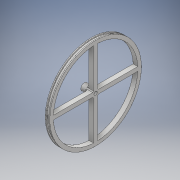
# Autodesk Inventor part: mtv_pushingWheel_2-25
Saved by Autodesk Inventor 2018 (Build 220112000, 112)
## iProperties
Created: 2019-02-07
Part Number: mtv_pushingWheel_2-25
Material: Generic
Document SubType Name: Modeling
Designer: Aditya Kendre
Density: 1 g/cm^3
Appearance: Default
Author: Aditya Kendre
Autodesk Inventor part; units mm, degrees
ref_plane "YZ Plane" through (0, 0, 0) normal (1, 0, 0) x (0, 1, 0)
ref_plane "XZ Plane" through (0, 0, 0) normal (0, 1, 0) x (-1, 0, 0)
ref_plane "XY Plane" through (0, 0, 0) normal (0, 0, 1) x (1, 0, 0)
sketch "Sketch1" plane through (0, 0, 0) normal (1, 0, 0) x (0, 1, 0)
  circle A0 centre (0, 0) radius 44
  dimension "d0" = 88
  constraints: 1 centre point, 1 coincident
  measures "d0" diameter of A0
extrude "Extrusion1" add sketch "Sketch1" along normal blind 3.5
sketch "Sketch2" plane through (3.5, 0, 0) normal (1, 0, 0) x (0, 0, -1)
  circle A0 centre (0, 0) radius 45
  dimension "d3" = 90
  constraints: 1 centre point, 1 coincident
  measures "d3" diameter of A0
extrude "Extrusion2" add sketch "Sketch2" along normal blind 1
sketch "Sketch3" plane through (0, 0, 0) normal (-1, 0, 0) x (0, 0, 1)
  circle A0 centre (0, 0) radius 45
  dimension "d6" = 90
  constraints: 1 centre point, 1 coincident
  measures "d6" diameter of A0
extrude "Extrusion3" add sketch "Sketch3" along normal blind 1
sketch "Sketch4" plane through (4.5, 0, 0) normal (1, 0, 0) x (0, 0, -1)
  circle A0 centre (0, 0) radius 41.5
  dimension "d9" = 83
  constraints: 1 centre point, 1 coincident
  measures "d9" diameter of A0
extrude "Extrusion4" cut sketch "Sketch4" against normal blind 6
sketch "Sketch5" plane through (4.5, 0, 0) normal (1, 0, 0) x (0, 0, -1)
  circle A0 centre (0, 0) radius 3.5
  dimension "d12" = 7
  constraints: 1 centre point, 1 coincident
  measures "d12" diameter of A0
extrude "Extrusion5" add sketch "Sketch5" against normal blind 10
sketch "Sketch6" plane through (4.5, 0, 0) normal (1, 0, 0) x (0, 0, -1)
  circle A0 centre (0, 0) radius 45
  constraints: 1 centre point, 1 coincident
extrude "Extrusion6" cut sketch "Sketch6" against normal blind 2
sketch "Sketch7" plane through (2.5, 0, 0) normal (1, 0, 0) x (0, 0, -1)
  circle A0 centre (0, 0) radius 3.5 projected
  circle A1 centre (0, 0) radius 41.5
  circle A2 centre (0, 0) radius 45
  constraints: 2 centre point, 2 coincident
extrude "Extrusion7" add sketch "Sketch7" along normal blind 1 contours A2
sketch "Sketch8" plane through (2.5, 0, 0) normal (1, 0, 0) x (0, 0, -1)
  circle A0 centre (0, 0) radius 3.5
  constraints: 1 centre point, 1 coincident
extrude "Extrusion8" add sketch "Sketch8" along normal blind 1
sketch "Sketch9" plane through (3.5, 0, 0) normal (1, 0, 0) x (0, 0, -1)
  circle A0 centre (0, 0) radius 1.625
  dimension "d21" = 3.25
  constraints: 1 centre point, 1 coincident
  measures "d21" diameter of A0
extrude "Extrusion9" cut sketch "Sketch9" against normal blind 10
sketch "Sketch10" plane through (3.5, 0, 0) normal (1, 0, 0) x (0, 0, -1)
  line L0 (2, 2.1756) -> (-2, 2.1756)
  line L1 (-2, 2.1756) -> (-2, 42.8244)
  line L2 (-2, 42.8244) -> (2, 42.8244)
  line L3 (2, 42.8244) -> (2, 2.1756)
  line L4 (2, 2.1756) -> (-2, 42.8244) construction
  line L5 (-2, 2.1756) -> (2, 42.8244) construction
  point P0 (0, 0)
  point P1 (0, 22.5)
  dimension "d24" = 4
  constraints: 12 end point, 2 midpoint, 2 parallel, 1 horizontal, 1 perpendicular
  measures "d24" distance of L1.end L2.end
extrude "Extrusion10" add sketch "Sketch10" against normal blind 4.5
pattern_circular "Circular Pattern1" count 4 over 360 about axis through (4.5, 0, 0) along (-1, 0, 0) of "Extrusion10"
fillet "Fillet1" radius 2 5 edges at (-1, 0, 3.5) (-1, -3.5, 0) (-1, 3.5, 0) (-1, -1.0481, -3.3394) (-1, 1.0481, -3.3394)
sketch "Sketch11" plane through (-5.5, 0, 0) normal (-1, 0, 0) x (0, 0, 1)
  circle A0 centre (0, 0) radius 1.625
  circle A1 centre (0, 0) radius 3.5
  constraints: 2 centre point, 2 coincident
extrude "Extrusion11" add sketch "Sketch11" along normal blind 2
sketch "Sketch12" plane through (-7.5, 0, 0) normal (-1, 0, 0) x (0, 0, 1)
  circle A0 centre (0, 0) radius 1.625
  circle A1 centre (0, 0) radius 2
  dimension "d33" = 4
  constraints: 2 centre point, 2 coincident
  measures "d33" diameter of A1
extrude "Extrusion12" add sketch "Sketch12" along normal blind 3.3
sketch "Sketch13" plane through (-10.8, 0, 0) normal (-1, 0, 0) x (0, 0, 1)
  circle A0 centre (0, 0) radius 3.5 projected
  line L0 (2.5211, -2.4277) -> (-2.5211, -2.4277)
  line L1 (-2.5211, -2.4277) -> (-2.5211, 2.4277)
  line L2 (-2.5211, 2.4277) -> (2.5211, 2.4277)
  line L3 (2.5211, 2.4277) -> (2.5211, -2.4277)
  line L4 (2.5211, -2.4277) -> (-2.5211, 2.4277) construction
  line L5 (-2.5211, -2.4277) -> (2.5211, 2.4277) construction
  constraints: 12 end point, 2 midpoint, 2 parallel, 1 horizontal, 1 perpendicular, 1 point on circle
extrude "Extrusion13" cut sketch "Sketch13" against normal blind 3.3 contours L3 L0 L1 L2
body "Solid1"
